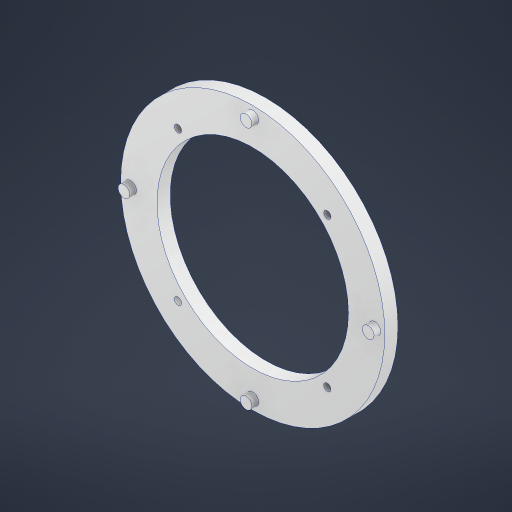
# Autodesk Inventor part: drehkranz
Saved by Autodesk Inventor 2023 (Build 270158000, 158)
## iProperties
Created: 2026-03-19
Part Number: drehkranz
Material: Aluminium 6061
Document SubType Name: Modeling
Designer: lerat
Mass: 719.664 g
Surface Area: 503.692 cm^2
Volume: 266.542 cm^3
Density: 2.7 g/cm^3
Appearance: Aluminium - flach
Author: lerat
Autodesk Inventor part; units mm, degrees
ref_plane "YZ Plane" through (0, 0, 0) normal (1, 0, 0) x (0, 1, 0)
ref_plane "XZ Plane" through (0, 0, 0) normal (0, 1, 0) x (-1, 0, 0)
ref_plane "XY Plane" through (0, 0, 0) normal (0, 0, 1) x (1, 0, 0)
sketch "Skizze1" plane through (0, 0, 0) normal (0, 0, 1) x (1, 0, 0)
  circle A0 centre (0, 0) radius 100
  circle A1 centre (0, 0) radius 72.5
  circle A2 centre (0, 0) radius 80 construction
  line L0 (0, 0) -> (-56.5685, 56.5685) construction
  line L1 (0, 0) -> (0, 80)
  circle A3 centre (-56.5685, 56.5685) radius 2.75
  circle A4 centre (-56.5685, -56.5685) radius 2.75
  circle A5 centre (56.5685, -56.5685) radius 2.75
  circle A6 centre (56.5685, 56.5685) radius 2.75
  dimension "d0" = 200
  dimension "d1" = 145
  dimension "d3" = 45
  dimension "d4" = 5.5
  dimension "d5" = 160
  dimension "d8" = 360
  constraints: 7 centre point, 4 end point, 3 coincident, 2 point on circle, 1 vertical, 9 other
  measures "d0" diameter of A0
  measures "d1" diameter of A1
  measures "d3" angle of L1 L0
  measures "d4" diameter of A3
  measures "d5" diameter of A2
extrude "Extrusion1" add sketch "Skizze1" along normal blind 10
sketch "Skizze2" plane through (0, 0, 10) normal (0, 0, 1) x (1, 0, 0)
  circle A0 centre (0, -92.5) radius 4.5
  point P0 (0, 0)
  dimension "d12" = 9
  dimension "d13" = 92.5
  constraints: 1 centre point, 1 vertical alignment
  measures "d12" diameter of A0
  measures "d13" distance of A0.centre point (0, 0)
extrude "Extrusion2" add sketch "Skizze2" along normal blind 5
pattern_circular "Runde Anordnung1" count 4 over 360 about axis through (0, 0, 0) along (0, 0, 1) of "Extrusion2"
sketch "Skizze3" plane through (0, 0, 0) normal (0, 0, -1) x (-1, 0, 0)
  circle A0 centre (-92.5, 0) radius 4.5 projected
  circle A1 centre (-92.5, 0) radius 2.5
  point P0 (0, 0)
  dimension "d19" = 5
  constraints: 1 centre point, 1 coincident
  measures "d19" diameter of A1
extrude "Extrusion3" cut sketch "Skizze3" against normal blind 5 contours A1
pattern_circular "Runde Anordnung2" count 4 over 360 about axis through (0, 0, 0) along (0, 0, 1) of "Extrusion3"
